Autodesk Inventor part; units mm, degrees
(part 2 of 2)
  spline S243 degree 2 poles (7.8662, -35.052) (8.1398, -34.9927) (8.6647, -34.7906) (8.8218, -34.7186) knots 0 0 0 1 2 2 2
  line L268 (8.8218, -34.7186) -> (9.3761, -37.2775)
  line L269 (9.3761, -37.2775) -> (6.6522, -37.8675)
  line L270 (6.6522, -37.8675) -> (6.5259, -37.2841)
  line L271 (6.5259, -37.2841) -> (8.61, -36.8327)
  line L272 (8.61, -36.8327) -> (8.3233, -35.509)
  spline S244 degree 2 poles (8.3233, -35.509) (8.2061, -35.5512) (7.9753, -35.6138) (7.8787, -35.6347) knots 0 0 0 1 2 2 2
  spline S245 degree 2 poles (7.8787, -35.6347) (7.4965, -35.7175) (6.9424, -35.707) (6.661, -35.5742) knots 0 0 0 1 2 2 2
  spline S246 degree 2 poles (6.661, -35.5742) (6.3754, -35.4423) (5.9879, -34.9365) (5.8903, -34.4859) knots 0 0 0 1 2 2 2
  line L273 (2.5129, -33.274) -> (2.6758, -38.3514)
  line L274 (2.6758, -38.3514) -> (-0.5007, -38.4533)
  line L275 (-0.5007, -38.4533) -> (-0.5199, -37.8526)
  line L276 (-0.5199, -37.8526) -> (1.9817, -37.7723)
  line L277 (1.9817, -37.7723) -> (1.9371, -36.3816)
  line L278 (1.9371, -36.3816) -> (-0.3958, -36.4564)
  line L279 (-0.3958, -36.4564) -> (-0.4151, -35.8557)
  line L280 (-0.4151, -35.8557) -> (1.9179, -35.7809)
  line L281 (1.9179, -35.7809) -> (1.8574, -33.8964)
  line L282 (1.8574, -33.8964) -> (-0.6442, -33.9767)
  line L283 (-0.6442, -33.9767) -> (-0.6635, -33.3759)
  line L284 (-0.6635, -33.3759) -> (2.5129, -33.274)
  line L285 (-4.304, -33.102) -> (-3.5202, -33.1636)
  line L286 (-3.5202, -33.1636) -> (-2.709, -34.6644)
  line L287 (-2.709, -34.6644) -> (-1.6487, -33.3108)
  line L288 (-1.6487, -33.3108) -> (-0.9223, -33.3679)
  line L289 (-0.9223, -33.3679) -> (-2.3878, -35.148)
  line L290 (-2.3878, -35.148) -> (-1.2334, -37.1672)
  line L291 (-1.2334, -37.1672) -> (-2.0173, -37.1056)
  line L292 (-2.0173, -37.1056) -> (-2.8253, -35.6174)
  line L293 (-2.8253, -35.6174) -> (-3.8764, -36.9594)
  line L294 (-3.8764, -36.9594) -> (-4.6028, -36.9023)
  line L295 (-4.6028, -36.9023) -> (-3.1462, -35.1297)
  line L296 (-3.1462, -35.1297) -> (-4.304, -33.102)
  spline S247 degree 2 poles (-11.5278, -34.0388) (-11.3444, -33.3676) (-10.5053, -32.4361) (-9.9662, -32.259) knots 0 0 0 1 2 2 2
  spline S248 degree 2 poles (-9.9662, -32.259) (-9.5289, -32.1267) (-8.7191, -32.1772) (-8.1234, -32.3399) knots 0 0 0 1 2 2 2
  line L297 (-8.1234, -32.3399) -> (-6.9956, -32.648)
  line L298 (-6.9956, -32.648) -> (-8.3342, -37.5484)
  line L299 (-8.3342, -37.5484) -> (-9.4501, -37.2436)
  spline S249 degree 2 poles (-9.4501, -37.2436) (-10.1411, -37.0549) (-10.871, -36.6336) (-11.099, -36.375) knots 0 0 0 1 2 2 2
  spline S250 degree 2 poles (-11.099, -36.375) (-11.4859, -35.9322) (-11.723, -34.7536) (-11.5278, -34.0388) knots 0 0 0 1 2 2 2
  spline S251 degree 2 poles (-10.8509, -34.2322) (-11.0049, -34.7961) (-10.8496, -35.6963) (-10.5421, -36.0235) knots 0 0 0 1 2 2 2
  spline S252 degree 2 poles (-10.5421, -36.0235) (-10.3223, -36.25) (-9.7686, -36.5506) (-9.3278, -36.671) knots 0 0 0 1 2 2 2
  line L300 (-9.3278, -36.671) -> (-8.8314, -36.8066)
  line L301 (-8.8314, -36.8066) -> (-7.8009, -33.034)
  line L302 (-7.8009, -33.034) -> (-8.2973, -32.8984)
  spline S253 degree 2 poles (-8.2973, -32.8984) (-8.7301, -32.7802) (-9.4234, -32.7402) (-9.7404, -32.8541) knots 0 0 0 1 2 2 2
  spline S254 degree 2 poles (-9.7404, -32.8541) (-10.1448, -32.9912) (-10.6946, -33.6603) (-10.8509, -34.2322) knots 0 0 0 1 2 2 2
  line L303 (-12.0927, -31.0686) -> (-11.492, -31.2958)
  line L304 (-11.492, -31.2958) -> (-12.8404, -34.8614)
  line L305 (-12.8404, -34.8614) -> (-13.4411, -34.6342)
  line L306 (-13.4411, -34.6342) -> (-12.0927, -31.0686)
  line L307 (-13.7077, -35.2112) -> (-13.0262, -35.4689)
  line L308 (-13.0262, -35.4689) -> (-13.2621, -36.0927)
  line L309 (-13.2621, -36.0927) -> (-13.9436, -35.835)
  line L310 (-13.9436, -35.835) -> (-13.7077, -35.2112)
  spline S255 degree 2 poles (-15.069, -30.1985) (-14.9736, -30.1797) (-14.6476, -30.1058) (-14.5095, -30.1026) knots 0 0 0 1 2 2 2
  spline S256 degree 2 poles (-14.5095, -30.1026) (-14.3182, -30.0927) (-13.9911, -30.1422) (-13.7305, -30.265) knots 0 0 0 1 2 2 2
  spline S257 degree 2 poles (-13.7305, -30.265) (-13.5182, -30.3651) (-13.2101, -30.706) (-13.1334, -30.9197) knots 0 0 0 1 2 2 2
  spline S258 degree 2 poles (-13.1334, -30.9197) (-13.0623, -31.1261) (-13.0913, -31.6222) (-13.2001, -31.853) knots 0 0 0 1 2 2 2
  spline S259 degree 2 poles (-13.2001, -31.853) (-13.3686, -32.2105) (-13.9089, -32.5748) (-14.3051, -32.5655) knots 0 0 0 1 2 2 2
  spline S260 degree 2 poles (-14.3051, -32.5655) (-14.6587, -32.5627) (-15.4956, -32.2911) (-15.9659, -32.1013) knots 0 0 0 1 2 2 2
  line L311 (-15.9659, -32.1013) -> (-16.0185, -32.213)
  spline S261 degree 2 poles (-16.0185, -32.213) (-16.1133, -32.4141) (-16.108, -32.7215) (-16.0296, -32.8449) knots 0 0 0 1 2 2 2
  spline S262 degree 2 poles (-16.0296, -32.8449) (-15.9513, -32.9683) (-15.6521, -33.164) (-15.4808, -33.2447) knots 0 0 0 1 2 2 2
  spline S263 degree 2 poles (-15.4808, -33.2447) (-15.2797, -33.3395) (-14.6799, -33.4766) (-14.3536, -33.4893) knots 0 0 0 1 2 2 2
  line L312 (-14.3536, -33.4893) -> (-14.3201, -33.5051)
  line L313 (-14.3201, -33.5051) -> (-14.5992, -34.0972)
  spline S264 degree 2 poles (-14.5992, -34.0972) (-14.7804, -34.0664) (-15.4326, -33.8955) (-15.7267, -33.7568) knots 0 0 0 1 2 2 2
  spline S265 degree 2 poles (-15.7267, -33.7568) (-16.0842, -33.5883) (-16.5194, -33.2467) (-16.6446, -33.0102) knots 0 0 0 1 2 2 2
  spline S266 degree 2 poles (-16.6446, -33.0102) (-16.7678, -32.7792) (-16.7416, -32.2409) (-16.5889, -31.9169) knots 0 0 0 1 2 2 2
  line L314 (-16.5889, -31.9169) -> (-15.4779, -29.5597)
  line L315 (-15.4779, -29.5597) -> (-14.897, -29.8335)
  line L316 (-14.897, -29.8335) -> (-15.069, -30.1985)
  line L317 (-15.2971, -30.6826) -> (-15.7482, -31.6396)
  spline S267 degree 2 poles (-15.7482, -31.6396) (-15.5309, -31.7192) (-14.8718, -31.9526) (-14.6463, -31.986) knots 0 0 0 1 2 2 2
  spline S268 degree 2 poles (-14.6463, -31.986) (-14.3821, -32.0241) (-13.9418, -31.8721) (-13.8189, -31.6114) knots 0 0 0 1 2 2 2
  spline S269 degree 2 poles (-13.8189, -31.6114) (-13.6785, -31.3135) (-13.8715, -30.8539) (-14.1917, -30.703) knots 0 0 0 1 2 2 2
  spline S270 degree 2 poles (-14.1917, -30.703) (-14.4636, -30.5748) (-15.021, -30.5988) (-15.2971, -30.6826) knots 0 0 0 1 2 2 2
  line L318 (-19.9062, -26.8062) -> (-21.1213, -28.648)
  spline S271 degree 2 poles (-21.1213, -28.648) (-21.2664, -28.8679) (-21.4792, -29.2651) (-21.4922, -29.4045) knots 0 0 0 1 2 2 2
  spline S272 degree 2 poles (-21.4922, -29.4045) (-21.512, -29.5542) (-21.3749, -29.8024) (-21.1928, -29.9226) knots 0 0 0 1 2 2 2
  spline S273 degree 2 poles (-21.1928, -29.9226) (-21.0279, -30.0314) (-20.5161, -30.078) (-20.1899, -30.0171) knots 0 0 0 1 2 2 2
  spline S274 degree 2 poles (-20.1899, -30.0171) (-20.1616, -29.9667) (-20.08, -29.8281) (-20.0211, -29.7388) knots 0 0 0 1 2 2 2
  line L319 (-20.0211, -29.7388) -> (-18.6383, -27.6427)
  line L320 (-18.6383, -27.6427) -> (-18.1022, -27.9963)
  line L321 (-18.1022, -27.9963) -> (-19.3173, -29.8382)
  spline S275 degree 2 poles (-19.3173, -29.8382) (-19.4624, -30.0581) (-19.6751, -30.4553) (-19.6881, -30.5947) knots 0 0 0 1 2 2 2
  spline S276 degree 2 poles (-19.6881, -30.5947) (-19.708, -30.7443) (-19.5709, -30.9926) (-19.3888, -31.1127) knots 0 0 0 1 2 2 2
  spline S277 degree 2 poles (-19.3888, -31.1127) (-19.217, -31.2261) (-18.6927, -31.2612) (-18.403, -31.2107) knots 0 0 0 1 2 2 2
  line L322 (-18.403, -31.2107) -> (-16.8342, -28.8328)
  line L323 (-16.8342, -28.8328) -> (-16.2981, -29.1865)
  line L324 (-16.2981, -29.1865) -> (-18.3974, -32.3685)
  line L325 (-18.3974, -32.3685) -> (-18.9334, -32.0148)
  line L326 (-18.9334, -32.0148) -> (-18.7022, -31.6643)
  spline S278 degree 2 poles (-18.7022, -31.6643) (-19.0501, -31.7356) (-19.6143, -31.6938) (-19.8617, -31.5306) knots 0 0 0 1 2 2 2
  spline S279 degree 2 poles (-19.8617, -31.5306) (-20.1435, -31.3447) (-20.4099, -30.7991) (-20.3306, -30.4322) knots 0 0 0 1 2 2 2
  spline S280 degree 2 poles (-20.3306, -30.4322) (-20.7537, -30.5427) (-21.3978, -30.5173) (-21.6658, -30.3405) knots 0 0 0 1 2 2 2
  spline S281 degree 2 poles (-21.6658, -30.3405) (-21.872, -30.2044) (-22.1248, -29.8551) (-22.1533, -29.6292) knots 0 0 0 1 2 2 2
  spline S282 degree 2 poles (-22.1533, -29.6292) (-22.1853, -29.401) (-22.0405, -28.8751) (-21.8252, -28.5486) knots 0 0 0 1 2 2 2
  line L327 (-21.8252, -28.5486) -> (-20.4423, -26.4525)
  line L328 (-20.4423, -26.4525) -> (-19.9062, -26.8062)
  line L329 (-21.9885, -25.0611) -> (-21.3693, -25.5912)
  line L330 (-21.3693, -25.5912) -> (-22.0011, -26.3292)
  line L331 (-22.0011, -26.3292) -> (-22.6203, -25.7992)
  line L332 (-22.6203, -25.7992) -> (-21.9885, -25.0611)
  line L333 (-23.8357, -27.219) -> (-23.2165, -27.7491)
  line L334 (-23.2165, -27.7491) -> (-23.8482, -28.4871)
  line L335 (-23.8482, -28.4871) -> (-24.4675, -27.9571)
  line L336 (-24.4675, -27.9571) -> (-23.8357, -27.219)
  spline S283 degree 2 poles (-28.8283, -24.6593) (-28.7085, -24.8006) (-28.4025, -25.0215) (-28.2347, -25.1113) knots 0 0 0 1 2 2 2
  spline S284 degree 2 poles (-28.2347, -25.1113) (-28.0748, -25.1916) (-27.8047, -25.281) (-27.6932, -25.3106) knots 0 0 0 1 2 2 2
  line L337 (-27.6932, -25.3106) -> (-27.6666, -25.342)
  line L338 (-27.6666, -25.342) -> (-28.2161, -25.8079)
  spline S285 degree 2 poles (-28.2161, -25.8079) (-28.4509, -25.7156) (-29.091, -25.2598) (-29.312, -24.9992) knots 0 0 0 1 2 2 2
  spline S286 degree 2 poles (-29.312, -24.9992) (-29.5356, -24.7355) (-29.7616, -24.2524) (-29.7844, -23.9965) knots 0 0 0 1 2 2 2
  spline S287 degree 2 poles (-29.7844, -23.9965) (-29.8057, -23.7231) (-29.6, -23.2464) (-29.3613, -23.0441) knots 0 0 0 1 2 2 2
  spline S288 degree 2 poles (-29.3613, -23.0441) (-29.0411, -22.7725) (-28.2008, -22.7833) (-27.8877, -23.0252) knots 0 0 0 1 2 2 2
  line L339 (-27.8877, -23.0252) -> (-27.85, -22.9932)
  spline S289 degree 2 poles (-27.85, -22.9932) (-27.9287, -22.8495) (-28.0526, -22.4742) (-28.0408, -22.259) knots 0 0 0 1 2 2 2
  spline S290 degree 2 poles (-28.0408, -22.259) (-28.032, -22.0465) (-27.8082, -21.5976) (-27.5538, -21.382) knots 0 0 0 1 2 2 2
  spline S291 degree 2 poles (-27.5538, -21.382) (-27.2932, -21.161) (-26.6987, -20.9646) (-26.3907, -20.9841) knots 0 0 0 1 2 2 2
  spline S292 degree 2 poles (-26.3907, -20.9841) (-26.0711, -21.0045) (-25.4817, -21.3305) (-25.2234, -21.6351) knots 0 0 0 1 2 2 2
  spline S293 degree 2 poles (-25.2234, -21.6351) (-24.9758, -21.9271) (-24.6326, -22.6184) (-24.5649, -22.8956) knots 0 0 0 1 2 2 2
  line L340 (-24.5649, -22.8956) -> (-25.1144, -23.3615)
  line L341 (-25.1144, -23.3615) -> (-25.1463, -23.3238)
  spline S294 degree 2 poles (-25.1463, -23.3238) (-25.1654, -23.0594) (-25.4142, -22.3204) (-25.6458, -22.0472) knots 0 0 0 1 2 2 2
  spline S295 degree 2 poles (-25.6458, -22.0472) (-25.7816, -21.8871) (-26.1536, -21.652) (-26.3603, -21.6438) knots 0 0 0 1 2 2 2
  spline S296 degree 2 poles (-26.3603, -21.6438) (-26.5644, -21.6386) (-26.9339, -21.763) (-27.1442, -21.9414) knots 0 0 0 1 2 2 2
  spline S297 degree 2 poles (-27.1442, -21.9414) (-27.3546, -22.1198) (-27.524, -22.4739) (-27.5093, -22.6503) knots 0 0 0 1 2 2 2
  spline S298 degree 2 poles (-27.5093, -22.6503) (-27.4946, -22.8268) (-27.3013, -23.1757) (-27.1522, -23.3515) knots 0 0 0 1 2 2 2
  line L342 (-27.1522, -23.3515) -> (-26.9659, -23.5713)
  line L343 (-26.9659, -23.5713) -> (-27.396, -23.936)
  line L344 (-27.396, -23.936) -> (-27.5425, -23.7633)
  spline S299 degree 2 poles (-27.5425, -23.7633) (-27.838, -23.4148) (-28.5435, -23.2574) (-28.8607, -23.5263) knots 0 0 0 1 2 2 2
  spline S300 degree 2 poles (-28.8607, -23.5263) (-29.0083, -23.6514) (-29.1228, -23.9429) (-29.1084, -24.0872) knots 0 0 0 1 2 2 2
  spline S301 degree 2 poles (-29.1084, -24.0872) (-29.0918, -24.2404) (-28.9428, -24.5243) (-28.8283, -24.6593) knots 0 0 0 1 2 2 2
  line L345 (-27.4726, -18.8893) -> (-27.0027, -19.5553)
  line L346 (-27.0027, -19.5553) -> (-27.7966, -20.1154)
  line L347 (-27.7966, -20.1154) -> (-28.2665, -19.4494)
  line L348 (-28.2665, -19.4494) -> (-27.4726, -18.8893)
  spline S302 degree 2 poles (-31.0082, -16.2007) (-30.6913, -16.0169) (-30.0323, -15.9059) (-29.7255, -15.9754) knots 0 0 0 1 2 2 2
  spline S303 degree 2 poles (-29.7255, -15.9754) (-29.4186, -16.0449) (-28.867, -16.4626) (-28.6687, -16.8045) knots 0 0 0 1 2 2 2
  spline S304 degree 2 poles (-28.6687, -16.8045) (-28.487, -17.1179) (-28.2706, -17.8109) (-28.2509, -18.0993) knots 0 0 0 1 2 2 2
  line L349 (-28.2509, -18.0993) -> (-28.874, -18.4607)
  line L350 (-28.874, -18.4607) -> (-28.8988, -18.418)
  spline S305 degree 2 poles (-28.8988, -18.418) (-28.8882, -18.3214) (-28.9067, -17.9942) (-28.9385, -17.8081) knots 0 0 0 1 2 2 2
  spline S306 degree 2 poles (-28.9385, -17.8081) (-28.9792, -17.5985) (-29.0788, -17.2708) (-29.1842, -17.0892) knots 0 0 0 1 2 2 2
  spline S307 degree 2 poles (-29.1842, -17.0892) (-29.2874, -16.9111) (-29.6098, -16.6507) (-29.8189, -16.6102) knots 0 0 0 1 2 2 2
  spline S308 degree 2 poles (-29.8189, -16.6102) (-30.0147, -16.5762) (-30.4298, -16.6647) (-30.6648, -16.801) knots 0 0 0 1 2 2 2
  spline S309 degree 2 poles (-30.6648, -16.801) (-30.8998, -16.9373) (-31.1246, -17.239) (-31.1541, -17.4179) knots 0 0 0 1 2 2 2
  spline S310 degree 2 poles (-31.1541, -17.4179) (-31.1922, -17.6066) (-31.0699, -18.0307) (-30.9398, -18.255) knots 0 0 0 1 2 2 2
  spline S311 degree 2 poles (-30.9398, -18.255) (-30.7994, -18.4972) (-30.4458, -18.9345) (-30.329, -19.0619) knots 0 0 0 1 2 2 2
  line L351 (-30.329, -19.0619) -> (-32.5938, -20.3756)
  line L352 (-32.5938, -20.3756) -> (-33.9922, -17.9648)
  line L353 (-33.9922, -17.9648) -> (-33.4758, -17.6653)
  line L354 (-33.4758, -17.6653) -> (-32.4059, -19.5099)
  line L355 (-32.4059, -19.5099) -> (-31.2343, -18.8303)
  spline S312 degree 2 poles (-31.2343, -18.8303) (-31.3105, -18.7318) (-31.441, -18.5314) (-31.4906, -18.446) knots 0 0 0 1 2 2 2
  spline S313 degree 2 poles (-31.4906, -18.446) (-31.6868, -18.1077) (-31.847, -17.5771) (-31.8071, -17.2685) knots 0 0 0 1 2 2 2
  spline S314 degree 2 poles (-31.8071, -17.2685) (-31.7693, -16.9562) (-31.4071, -16.432) (-31.0082, -16.2007) knots 0 0 0 1 2 2 2
  dimension "d30" = 66.675
  constraints: 1 centre point, 1 coincident, 1 other
  measures "d30" diameter of A0
extrude "TextExtrusion" cut sketch "Sketch5" against normal blind 1.27 contours L102 L103 L104 L105 | L110 L111 L112 L113 | L121 L122 S91 S92 S93 S94 S95 S96 L123 L124 S97 S98 S99 S100 S101 L125 L126 | L174 L175 S133 S134 S135 S136 S137 S138 L176 L177 S139 S140 S141 S142 S143 L178 L179 | L252 L253 L254 L255 L256 L257 S233 L258 L259 L260 L261 | L284 L273 L274 L275 L276 L277 L278 L279 L280 L281 L282 L283 | A0 L29 L30 L31 | S29 L44 L45 L46 L47 L48 L49 L50 L51 L52 L53 L54 S30 S31 S32 L55 L56 S33 A0 | A0 S33 S29 | S14 S15 A0 | A0 S15 S16 S17 S18 L21 S19 S20 S21 L22 L23 S22 S23 S24 L24 L25 L26 S13 S14 | S44 L68 L69 S45 S46 S47 S48 S49 L70 L71 L72 S50 S51 S52 S34 S35 L65 L66 S36 S37 S38 S39 L67 S40 S41 S42 S43 A0 | A0 S43 S44 | S12 S8 A0 | A0 S8 L8 L9 L10 L11 L12 L13 L14 L15 L16 L17 L18 S9 S10 S11 L19 L20 S12 | S53 S54 S55 S56 L85 L86 S57 S58 S59 L87 L88 S60 S61 A0 | A0 S61 S53 | S0 S1 A0 | A0 S1 S2 S3 S0 | A0 L0 L1 L2 L3 L4 L5 L6 | S67 S68 S69 S66 A0 | A0 S66 S67 | S303 S304 A0 | A0 S304 L349 L350 S305 S306 S307 S308 S309 S310 S311 L351 L352 L353 L354 L355 S312 S313 S314 S302 S303 | S80 L114 L115 S81 S82 S83 S84 S85 S86 S87 L116 L117 L118 L119 L120 S88 S89 S90 S78 S79 A0 | A0 S79 S80 | S292 S293 A0 | A0 S293 L340 L341 S294 S295 S296 S297 S298 L342 L343 L344 S299 S300 S301 S283 S284 L337 L338 S285 S286 S287 S288 L339 S289 S290 S291 S292 | A0 L321 S275 S276 S277 L322 L323 L324 L325 L326 S278 S279 S280 S281 S282 L327 L328 L318 S271 S272 S273 S274 L319 | S104 L127 L128 S105 S106 S107 S108 S109 S110 S111 L129 L130 L131 L132 L133 S112 S113 S114 S102 S103 A0 | A0 S103 S104 | S256 S257 A0 | A0 S257 S258 S259 S260 L311 S261 S262 S263 L312 L313 S264 S265 S266 L314 L315 L316 S255 S256 | S117 L134 L135 S118 S119 S120 S121 S122 S123 S124 L136 L137 L138 L139 L140 S125 S126 S127 S115 S116 A0 | A0 S116 S117 | A0 L304 L305 L306 | S128 L153 L154 L155 L156 L157 L158 L159 L160 L161 L162 L163 S129 S130 S131 L164 L165 S132 A0 | A0 S132 S128 | S235 S236 A0 | A0 S236 L266 L267 S237 S238 S239 S240 S241 S242 S243 L268 L269 L270 L271 L272 S244 S245 S246 S234 S235 | S146 L191 L192 S147 S148 S149 S150 S151 S152 S153 L193 L194 L195 L196 L197 S154 S155 S156 S144 S145 A0 | A0 S145 S146 | S157 L198 L199 S158 S159 S160 S161 S162 S163 S164 S165 L200 L201 S166 S167 S168 S169 S170 S171 S172 A0 | A0 S172 S157 | A0 L236 S225 S226 S227 L237 L238 L239 L240 L241 S228 S229 S230 S231 S232 L242 L243 L233 S221 S222 S223 S224 L234 | S206 S207 A0 | A0 S207 S208 S209 S210 L226 S211 S212 S213 L227 L228 S214 S215 S216 L229 L230 L231 S205 S206 | L204 L205 L206 S175 S176 S173 A0 S174 L202 | A0 L202 L203 L204 | A0 L219 L220 L221 | A0 S173 S174 | A0 L209 L210 L211 | S182 S183 S184 S181 A0 | A0 S181 S182 | S189 S190 A0 | A0 S190 S191 S192 S189 | L32 L33 L34 L35 L36 L37 L38 L39 L40 L41 L42 L43 | L57 L58 L59 L60 | L61 L62 L63 L64 | L73 L74 L75 L76 L77 L78 L79 L80 L81 L82 L83 L84 | L90 L91 L92 L93 L94 L95 L96 L97 L98 L99 L100 L101 | L106 L107 L108 L109 | L141 L142 L143 L144 L145 L146 L147 L148 L149 L150 L151 L152 | L166 L167 L168 L169 | L170 L171 L172 L173 | L180 L181 L182 L183 | L184 L185 L186 L187 L188 L189 L190 | S197 S198 L212 L213 L214 S199 S200 | L222 L223 L224 L225 | L244 L245 L246 L247 | L248 L249 L250 L251 | L262 L263 L264 L265 | L285 L286 L287 L288 L289 L290 L291 L292 L293 L294 L295 L296 | S247 S248 L297 L298 L299 S249 S250 | L307 L308 L309 L310 | L329 L330 L331 L332 | L333 L334 L335 L336 | L345 L346 L347 L348
chamfer "StringHoleChamfer" distance 3.175 angle 45 2 edges at (-16.6229, 48.8983, 9.3048) (16.6229, 15.8783, 9.3048)
chamfer "HexChamfer" distance 1.5875 angle 45 12 edges at (5.7467, 69.85, 3.3179) (0, 69.85, 6.6357) (-5.7467, 69.85, 3.3179) (0, 69.85, -6.6358) (5.7467, 69.85, -3.3179) (-5.7467, 69.85, -3.3179) (0, -6.35, 6.6357) (5.7467, -6.35, 3.3179) (5.7467, -6.35, -3.3179) (0, -6.35, -6.6358) (-5.7467, -6.35, -3.3179) (-5.7467, -6.35, 3.3179)
ref_plane "Work Plane1" through (0, 51.435, -19.05) normal (0, 0, 1) x (1, 0, 0)
sketch "Sketch8" plane through (0, 51.435, -19.05) normal (0, 0, 1) x (1, 0, 0)
  line L0 (-42.545, 14.605) -> (42.545, 14.605) projected
  line L1 (-42.545, -47.625) -> (42.545, -47.625) projected
  line L2 (0, -51.435) -> (0, 14.605) construction
  point P0 (0, 0)
  point P1 (0, -33.02)
  dimension "d42" = 14.605
  dimension "d43" = 14.605
  dimension "d51" = 0
  dimension "d52" = 0
  constraints: 2 end point, 1 midpoint
  measures "d42" distance from line of point (0, 0) L0
  measures "d43" distance from line of point (0, -33.02) L1
  measures "d51" distance from line of point (0, 0) L2
  measures "d52" distance from line of point (0, -33.02) L2
hole "#6 0.150 Insert" at (0, 51.435, -19.05) at (0, 18.415, -19.05) direction (0, 0, 1) diameter 3.8354 depth 12.7 counterbore diameter 4.8514 counterbore depth 3.81
equation "\"d0\" = spoolHeightWithoutSpacer"
equation "\"d1\" = supportChannels"
equation "\"d2\" = spoolInteriroRadius"
equation "\"d3\" = spoolExteriorRadius"
equation "\"d4\" = spoolFiletRadius"
equation "\"d5\" = spoolFiletRadius"
equation "\"d36\" = spacerDiameter"
equation "\"d37\" = spaceHeight"
equation "\"d8\" = hexDiameter"
equation "\"d17\" = holeCenter"
equation "\"d18\" = holeCenter"
equation "\"d19\" = holeForString"
equation "\"d20\" = stringHoleCenterFromHexShaft"
equation "\"d21\" = stringHoleCenterFromHexShaft"
equation "\"d30\" = textCircleDiameter"
equation "\"d31\" = textDepth"
equation "\"d33\" = stringHoleChamfer"
equation "\"d39\" = hexHoleChamfer"
equation "\"d42\" = holeCenter"
equation "\"d43\" = holeCenter"
equation "\"holeForString\" = stringDiameter + clearanceForString"
equation "\"stringDiameter\" = 3.048"
equation "\"clearanceForString\" = 2.032"
equation "\"spoolHeightWithoutSpacer\" = 69.85"
equation "\"hexShaftDiameter\" = 12.7"
equation "\"clearanceForHexShaft\" = 0.5715"
equation "\"hexDiameter\" = hexShaftDiameter + clearanceForHexShaft"
equation "\"supportChannels\" = 3.81"
equation "\"spoolInteriorDiameter\" = 38.1"
equation "\"spoolInteriroRadius\" = 0.5 * spoolInteriorDiameter"
equation "\"spoolExteriorDiameter\" = 88.9"
equation "\"spoolExteriorRadius\" = 0.5 * spoolExteriorDiameter"
equation "\"spoolFiletRadius\" = 0.5 * supportChannels"
equation "\"holeCenter\" = 0.25 * spoolHeightWithoutSpacer - 0.75 * supportChannels"
equation "\"hexHoleChamfer\" = 1.5875"
equation "\"stringHoleCenterFromHexShaft\" = 0.5 * hexDiameter + 0.5 * holeForString"
equation "\"textCircleDiameter\" = 0.75 * spoolExteriorDiameter"
equation "\"textHeight\" = 6.096"
equation "\"textDepth\" = 1.27"
equation "\"stringHoleChamfer\" = 3.175"
equation "\"spoolTotalHeight\" = 76.2"
equation "\"spaceHeight\" = spoolTotalHeight - spoolHeightWithoutSpacer"
equation "\"spacerDiameter\" = 24.13"
body "Solid1"
